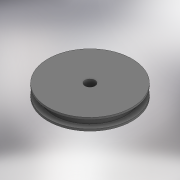
# Autodesk Inventor part: servo_pulley
Saved by Autodesk Inventor 2020 (Build 240168000, 168)
## iProperties
Created: 2020-06-18
Part Number: servo_pulley
Material: Generic
Document SubType Name: Modeling
Designer: pc-konvi
Density: 1 g/cm^3
Appearance: Gray
Author: pc-konvi
Autodesk Inventor part; units mm, degrees
ref_plane "YZ Plane" through (0, 0, 0) normal (1, 0, 0) x (0, 1, 0)
ref_plane "XZ Plane" through (0, 0, 0) normal (0, 1, 0) x (-1, 0, 0)
ref_plane "XY Plane" through (0, 0, 0) normal (0, 0, 1) x (1, 0, 0)
sketch "Sketch1" plane through (0, 0, 0) normal (0, 0, 1) x (1, 0, 0)
  line L0 (0, 0) -> (18, 0)
  line L1 (18, 0) -> (18, 3)
  line L2 (18, 3) -> (0, 3)
  line L3 (0, 3) -> (0, 0)
  line L4 (0, 3) -> (21, 3)
  line L5 (21, 3) -> (21, 2)
  line L6 (21, 2) -> (0, 2)
  line L7 (0, 2) -> (0, 3)
  point P0 (18, 2)
  dimension "d0" = 18
  dimension "d1" = 3
  dimension "d2" = 21
  dimension "d3" = 1
  constraints: 16 end point, 4 parallel, 2 horizontal, 2 perpendicular
  measures "d0" distance of L2.end L1.end
  measures "d1" distance of L1.end L0.end
  measures "d2" distance of L5.end L6.end
  measures "d3" distance of L4.end L5.end
revolve "Revolution1" add sketch "Sketch1" angle 360 about axis through (0, 3, 0) along (0, -1, 0)
mirror "Mirror1" about plane through (0, 0, 0) normal (0, 1, 0) of "Revolution1"
sketch "Sketch2" plane through (0, 3, 0) normal (0, 1, 0) x (1, 0, 0)
  circle A0 centre (0, 0) radius 2.5
  dimension "d5" = 5
  constraints: 1 centre point, 1 coincident
  measures "d5" diameter of A0
extrude "Extrusion1" cut sketch "Sketch2" against normal blind 10
body "Solid1"
